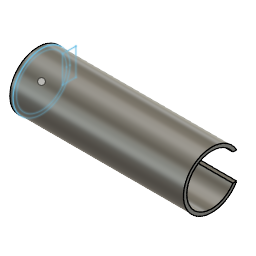
Battery Holder (Autodesk Fusion 360 design; units mm, degrees)
part number: 2026-06-09-18-26-14-445
Autodesk Fusion 360 part; units mm, degrees
note: some values were not read from the file. Set by a fixed rule: which sketch regions a step uses.
sketch "Sketch1" plane through (0, 0, 0) normal (1, 0, 0) x (0, 0, -1)
  circle A0 centre (10.5652, 11.0695) radius 8.5
  circle A1 centre (10.5652, 11.0695) radius 7.5
  line L0 (16.8789, 15.1175) -> (16.8789, 7.0215)
  line L1 (16.8789, 7.0215) -> (20.8789, 7.0215)
  line L2 (16.8789, 15.1175) -> (20.8789, 15.1175)
  line L3 (20.8789, 15.1175) -> (20.8789, 7.0215)
  dimension "d5" = 17
  dimension "d6" = 15
  dimension "d95" = 4
  dimension "d96" = 4
  constraint concentric A0 A1
  constraint coincident A1 L0.start
  constraint vertical L0
  constraint coincident A1 L0.end
  constraint perpendicular L0 L1
  constraint perpendicular L0 L2
  measures "d5" diameter of A0
  measures "d6" diameter of A1
  measures "d95" distance of L0.end L1.end
  measures "d96" distance of L0.start L2.end
extrude "Extrude14" add sketch "Sketch1" against normal blind 1 contours A0 A1 L1 L2 | A0 A1 L1 L2 | A1 L0 | A1 L0
extrude "Extrude15" add sketch "Sketch1" along normal blind 51 contours A0 A1 L1 L2 picked at (2.4358, 10.4711)
extrude "Extrude1" [suppressed]
extrude "Extrude2" [suppressed]
extrude "Extrude3" [suppressed]
sketch "Sketch2" plane through (0, 0, 0) normal (0, 0, 1) x (1, 0, 0)
  line L0 (50, 8, -2) -> (35, 8, -2)
  line L1 (35, 8, -2) -> (35, 13, -2)
  line L2 (35, 13, -2) -> (50, 13, -2)
  line L3 (50, 13, -2) -> (50, 8, -2)
  line L4 (35, 13, -2) -> (38, 13, -2)
  line L5 (38, 13, -2) -> (38, 15, -2)
  line L6 (38, 15, -2) -> (35, 15, -2)
  line L7 (35, 15, -2) -> (35, 13, -2)
  line L8 (35, 8, -2) -> (38, 8, -2)
  line L9 (38, 8, -2) -> (38, 6, -2)
  line L10 (38, 6, -2) -> (35, 6, -2)
  line L11 (35, 6, -2) -> (35, 8, -2)
  dimension "d14" = 2
  dimension "d15" = 2
  dimension "d16" = 3
  dimension "d17" = 3
  dimension "d18" = 5
  dimension "d19" = 15
extrude "Extrude4" [suppressed]
sketch "Sketch4" plane through (0, 0, 0) normal (0, 0, 1) x (1, 0, 0)
  line L0 (35.0001, 13, -23) -> (50.0001, 13, -23)
  line L1 (50.0001, 13, -23) -> (50.0001, 8, -23)
  line L2 (50.0001, 8, -23) -> (35.0001, 8, -23)
  line L3 (35.0001, 8, -23) -> (35.0001, 13, -23)
  line L4 (35.0001, 13, -23) -> (38.0001, 13, -23)
  line L5 (38.0001, 13, -23) -> (38.0001, 15, -23)
  line L6 (38.0001, 15, -23) -> (35.0001, 15, -23)
  line L7 (35.0001, 15, -23) -> (35.0001, 13, -23)
  line L8 (35.0001, 8, -23) -> (38.0001, 8, -23)
  line L9 (38.0001, 8, -23) -> (38.0001, 6, -23)
  line L10 (38.0001, 6, -23) -> (35.0001, 6, -23)
  line L11 (35.0001, 6, -23) -> (35.0001, 8, -23)
  dimension "d24" = 15
  dimension "d25" = 3
  dimension "d26" = 2
  dimension "d27" = 2
  dimension "d28" = 3
  dimension "d42" = 5
extrude "Extrude6" [suppressed]
sketch "Sketch5" plane through (0, 0, 0) normal (0, 1, 0) x (1, 0, 0)
  line L0 (50, 15, 2) -> (35, 15, 2)
  line L1 (35, 15, 2) -> (35, 10, 2)
  line L2 (35, 10, 2) -> (50, 10, 2)
  line L3 (50, 10, 2) -> (50, 15, 2)
  line L4 (35, 15, 2) -> (38, 15, 2)
  line L5 (38, 15, 2) -> (38, 17, 2)
  line L6 (38, 17, 2) -> (35, 17, 2)
  line L7 (35, 17, 2) -> (35, 15, 2)
  line L8 (35, 10, 2) -> (38, 10, 2)
  line L9 (38, 10, 2) -> (38, 8, 2)
  line L10 (38, 8, 2) -> (35, 8, 2)
  line L11 (35, 8, 2) -> (35, 10, 2)
  dimension "d31" = 15
  dimension "d32" = 5
  dimension "d33" = 3
  dimension "d34" = 2
  dimension "d35" = 3
  dimension "d36" = 2
extrude "Extrude7" [suppressed]
sketch "Sketch6" plane through (0, 0, 0) normal (1, 0, 0) x (0, 0, -1)
  line L0 (-30, 2) -> (-5, 2)
  line L1 (-5, 2) -> (-5, 17)
  line L2 (-5, 17) -> (-30, 17)
  line L3 (-30, 17) -> (-30, 2)
  line L4 (-30, 17) -> (-27.95, 17)
  line L5 (-27.95, 17) -> (-27.95, 14.9)
  line L6 (-27.95, 14.9) -> (-30, 14.9)
  line L7 (-30, 14.9) -> (-30, 17)
  line L8 (-27.95, 14.9) -> (-26.1, 14.9)
  line L9 (-26.1, 14.9) -> (-26.1, 10.3)
  line L10 (-26.1, 10.3) -> (-27.95, 10.3)
  line L11 (-27.95, 10.3) -> (-27.95, 14.9)
  line L12 (-5, 17) -> (-7.05, 17)
  line L13 (-7.05, 17) -> (-7.05, 14.9)
  line L14 (-7.05, 14.9) -> (-5, 14.9)
  line L15 (-5, 14.9) -> (-5, 17)
  line L16 (-7.05, 14.9) -> (-8.9, 14.9)
  line L17 (-8.9, 14.9) -> (-8.9, 10.3)
  line L18 (-8.9, 10.3) -> (-7.05, 10.3)
  line L19 (-7.05, 10.3) -> (-7.05, 14.9)
  line L20 (-30, 4) -> (-19.9, 4)
  line L21 (-19.9, 4) -> (-19.9, 2)
  line L22 (-19.9, 2) -> (-30, 2)
  line L23 (-30, 2) -> (-30, 4)
  line L24 (-19.9, 4) -> (-15.3, 4)
  line L25 (-15.3, 4) -> (-15.3, 5.85)
  line L26 (-15.3, 5.85) -> (-19.9, 5.85)
  line L27 (-19.9, 5.85) -> (-19.9, 4)
  line L28 (-5, 4) -> (-5, 1.95)
  line L29 (-5, 1.95) -> (-15.3, 1.95)
  line L30 (-15.3, 1.95) -> (-15.3, 4)
  line L31 (-27.025, 10.3) -> (-27.025, 12.05)
  line L32 (-27.025, 14.9) -> (-27.025, 13.15)
  line L33 (-27.95, 13.15) -> (-26.1, 13.15)
  line L34 (-27.95, 12.05) -> (-26.1, 12.05)
  line L35 (-7.975, 14.9) -> (-7.975, 13.15)
  line L36 (-7.975, 10.3) -> (-7.975, 12.05)
  line L37 (-7.05, 12.05) -> (-8.9, 12.05)
  line L38 (-7.05, 13.15) -> (-8.9, 13.15)
  line L39 (-19.9, 4.925) -> (-18.15, 4.925)
  line L40 (-18.15, 4) -> (-18.15, 5.85)
  line L41 (-15.3, 4.925) -> (-17.05, 4.925)
  line L42 (-17.05, 4) -> (-17.05, 5.85)
  dimension "d40" = 25
  dimension "d41" = 15
  dimension "d43" = 2.05
  dimension "d44" = 2.1
  dimension "d45" = 1.85
  dimension "d46" = 4.6
  dimension "d47" = 2.05
  dimension "d48" = 2.1
  dimension "d49" = 1.85
  dimension "d50" = 4.6
  dimension "d51" = 10.1
  dimension "d52" = 2
  dimension "d53" = 4.6
  dimension "d54" = 1.85
  dimension "d56" = 2.05
  dimension "d57" = 1.75
  dimension "d58" = 1.75
  dimension "d59" = 1.75
  dimension "d60" = 1.75
  dimension "d61" = 1.75
  dimension "d62" = 1.75
  constraint horizontal L0
  constraint vertical L1
  constraint horizontal L2
  constraint vertical L3
  constraint horizontal L4
  constraint vertical L5
  constraint horizontal L6
  constraint vertical L7
  constraint horizontal L8
  constraint vertical L9
  constraint horizontal L10
  constraint vertical L11
  constraint horizontal L12
  constraint vertical L13
  constraint horizontal L14
  constraint vertical L15
  constraint horizontal L16
  constraint vertical L17
  constraint horizontal L18
  constraint vertical L19
  constraint horizontal L20
  constraint vertical L21
  constraint horizontal L22
  constraint vertical L23
  constraint coincident L3 L20.start
  constraint horizontal L24
  constraint vertical L25
  constraint horizontal L26
  constraint vertical L27
  constraint horizontal L29
  constraint vertical L30
  constraint midpoint L10 L31.start
  constraint perpendicular L10 L31
  constraint vertical L32
  constraint midpoint L8 L32.start
  constraint coincident L11 L33.start
  constraint coincident L9 L33.end
  constraint perpendicular L9 L33
  constraint coincident L11 L34.start
  constraint coincident L9 L34.end
  constraint perpendicular L9 L34
  constraint midpoint L16 L35.start
  constraint perpendicular L16 L35
  constraint midpoint L18 L36.start
  constraint perpendicular L18 L36
  constraint coincident L19 L37.start
  constraint coincident L17 L37.end
  constraint perpendicular L17 L37
  constraint coincident L19 L38.start
  constraint coincident L17 L38.end
  constraint perpendicular L17 L38
  constraint midpoint L27 L39.start
  constraint perpendicular L27 L39
  constraint coincident L24 L40.start
  constraint coincident L26 L40.end
  constraint perpendicular L26 L40
  constraint midpoint L25 L41.start
  constraint perpendicular L25 L41
  constraint coincident L24 L42.start
  constraint coincident L26 L42.end
  constraint perpendicular L26 L42
  measures "d40" distance of L0.start L0.end
  measures "d41" distance of L0.start L2.end
  measures "d43" distance of L2.end L4.end
  measures "d44" distance of L2.end L6.end
  measures "d45" distance of L5.end L8.end
  measures "d46" distance of L5.end L10.end
  measures "d47" distance of L1.end L12.end
  measures "d48" distance of L1.end L14.end
  measures "d49" distance of L13.end L16.end
  measures "d50" distance of L13.end L18.end
  measures "d51" distance of L20.start L20.end
  measures "d52" distance of L20.start L0.start
  measures "d53" distance of L20.end L24.end
  measures "d54" distance of L20.end L26.end
  measures "d56" distance of L24.end L29.end
  measures "d57" distance of L31.start L31.end
  measures "d58" distance of L32.start L32.end
  measures "d59" distance of L35.start L35.end
  measures "d60" distance of L36.start L36.end
  measures "d61" distance of L39.start L39.end
  measures "d62" distance of L41.start L41.end
sketch "Sketch7" plane through (0, 0, 0) normal (1, 0, 0) x (0, 0, -1)
extrude "Extrude8" [suppressed]
extrude "Extrude9" [suppressed]
extrude "Extrude10" [suppressed]
sketch "Sketch8" plane through (0, 14.9, 0) normal (0, 1, 0) x (-1, 0, 0)
  line L0 (0, 26.1) -> (0, 27.95)
  line L1 (0, 27.95) -> (-14.5, 27.95)
  line L2 (-14.5, 27.95) -> (-14.5, 26.1)
  line L3 (-14.5, 26.1) -> (0, 26.1)
  line L4 (-14.5, 26.1) -> (-12.3, 26.1)
  line L5 (-12.3, 26.1) -> (-12.3, 27.95)
  line L6 (-12.3, 27.95) -> (-14.5, 27.95)
  line L7 (-14.5, 27.95) -> (-14.5, 26.1)
  dimension "d69" = 2.2
  constraint horizontal L4
  constraint vertical L5
  constraint horizontal L6
  constraint vertical L7
  constraint coincident L2.end L3.start
  measures "d69" distance of L2.end L4.end
sketch "Sketch9" plane through (0, 0, 27.95) normal (0, 0, 1) x (1, 0, 0)
  line L0 (0, 14.9) -> (0, 10.3)
  line L1 (0, 10.3) -> (14.5, 10.3)
  line L2 (14.5, 10.3) -> (14.5, 12.05)
  line L3 (14.5, 12.05) -> (7.5, 12.05)
  line L4 (7.5, 12.05) -> (7.5, 13.15)
  line L5 (7.5, 13.15) -> (14.5, 13.15)
  line L6 (14.5, 13.15) -> (14.5, 14.9)
  line L7 (14.5, 14.9) -> (0, 14.9)
  line L8 (14.5, 14.9) -> (12.3, 14.9)
  line L9 (12.3, 14.9) -> (12.3, 16.6)
  line L10 (12.3, 16.6) -> (14.5, 14.9)
  line L11 (14.5, 10.3) -> (12.3, 10.3)
  line L12 (12.3, 10.3) -> (12.3, 8.6)
  line L13 (12.3, 8.6) -> (14.5, 10.3)
  dimension "d70" = 2.2
  dimension "d71" = 1.7
  dimension "d72" = 2.2
  dimension "d73" = 1.7
  constraint coincident L6.end L7.start
  constraint perpendicular L6 L8
  constraint perpendicular L8 L9
  constraint coincident L1.end L2.start
  constraint perpendicular L2 L11
  constraint perpendicular L11 L12
  measures "d70" distance of L6.end L8.end
  measures "d71" distance of L8.end L9.end
  measures "d72" distance of L1.end L11.end
  measures "d73" distance of L11.end L12.end
extrude "Extrude11" [suppressed]
sketch "Sketch10" plane through (0, 0, 7.05) normal (0, 0, -1) x (-1, 0, 0)
  line L0 (0, 10.3) -> (0, 14.9)
  line L1 (0, 14.9) -> (-14.5, 14.9)
  line L2 (-14.5, 14.9) -> (-14.5, 13.15)
  line L3 (-14.5, 13.15) -> (-7.5, 13.15)
  line L4 (-7.5, 13.15) -> (-7.5, 12.05)
  line L5 (-7.5, 12.05) -> (-14.5, 12.05)
  line L6 (-14.5, 12.05) -> (-14.5, 10.3)
  line L7 (-14.5, 10.3) -> (0, 10.3)
  line L8 (-14.5, 14.9) -> (-12.3, 14.9)
  line L9 (-12.3, 14.9) -> (-12.3, 16.6)
  line L10 (-12.3, 16.6) -> (-14.5, 14.9)
  line L11 (-3.3943, 7.7424) -> (-3.3943, 7.4172)
  line L12 (-14.5, 10.3) -> (-12.3, 10.3)
  line L13 (-12.3, 10.3) -> (-12.3, 8.6)
  line L14 (-12.3, 8.6) -> (-14.5, 10.3)
  dimension "d76" = 2.2
  dimension "d77" = 1.7
  dimension "d78" = 2.2
  dimension "d79" = 1.7
  constraint coincident L1.end L2.start
  constraint perpendicular L2 L8
  constraint perpendicular L8 L9
  constraint perpendicular L7 L11
  constraint coincident L6.end L7.start
  constraint perpendicular L6 L12
  constraint perpendicular L12 L13
  measures "d76" distance of L1.end L8.end
  measures "d77" distance of L8.end L9.end
  measures "d78" distance of L6.end L12.end
  measures "d79" distance of L12.end L13.end
extrude "Extrude12" [suppressed]
sketch "Sketch11" plane through (0, 4, 0) normal (0, -1, 0) x (1, 0, 0)
  line L0 (0, 19.9) -> (0, 15.3)
  line L1 (0, 15.3) -> (14.5, 15.3)
  line L2 (14.5, 15.3) -> (14.5, 17.05)
  line L3 (14.5, 17.05) -> (7.5, 17.05)
  line L4 (7.5, 17.05) -> (7.5, 18.15)
  line L5 (7.5, 18.15) -> (14.5, 18.15)
  line L6 (14.5, 18.15) -> (14.5, 19.9)
  line L7 (14.5, 19.9) -> (0, 19.9)
  line L8 (14.5, 19.9) -> (12.3, 19.9)
  line L9 (12.3, 19.9) -> (12.3, 21.6)
  line L10 (12.3, 21.6) -> (14.5, 19.9)
  line L11 (14.5, 15.3) -> (12.3, 15.3)
  line L12 (12.3, 15.3) -> (12.3, 13.6)
  line L13 (14.5, 15.3) -> (12.3, 13.6)
  dimension "d82" = 2.2
  dimension "d83" = 1.7
  dimension "d84" = 2.2
  dimension "d85" = 1.7
  constraint coincident L6.end L7.start
  constraint perpendicular L6 L8
  constraint vertical L9
  constraint coincident L1.end L2.start
  constraint perpendicular L2 L11
  constraint perpendicular L1 L12
  measures "d82" distance of L6.end L8.end
  measures "d83" distance of L8.end L9.end
  measures "d84" distance of L1.end L11.end
  measures "d85" distance of L11.end L12.end
extrude "Extrude13" [suppressed]
extrude "Extrude5" [suppressed]
